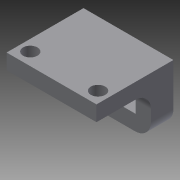
# Autodesk Inventor part: switch Holder
Saved by Autodesk Inventor 2014 (Build 180170000, 170)
## iProperties
Created: 2013-12-07
Part Number: switch Holder
Material: Generic
Document SubType Name: Modeling
Designer: Jesse Stevenson
Density: 1 g/cm^3
Appearance: Default
Author: Jesse Stevenson
Autodesk Inventor part; units mm, degrees
ref_plane "YZ Plane" through (0, 0, 0) normal (1, 0, 0) x (0, 1, 0)
ref_plane "XZ Plane" through (0, 0, 0) normal (0, 1, 0) x (-1, 0, 0)
ref_plane "XY Plane" through (0, 0, 0) normal (0, 0, 1) x (1, 0, 0)
sketch "Sketch1" plane through (0, 0, 0) normal (0, 0, 1) x (1, 0, 0)
  line L0 (0, 0) -> (29.2862, 0)
  line L1 (29.2862, 0) -> (29.2862, 13.716)
  line L2 (29.2862, 13.716) -> (0, 13.716)
  line L3 (0, 13.716) -> (0, 0)
  line L4 (14.6431, 13.716) -> (14.6431, 0) construction
  line L5 (0, 6.858) -> (29.2862, 6.858) construction
  line L6 (-7.62, -7.62) -> (36.9062, -7.62)
  line L7 (36.9062, -7.62) -> (36.9062, 21.336)
  line L8 (36.9062, 21.336) -> (-7.62, 21.336)
  line L9 (-7.62, 21.336) -> (-7.62, -7.62)
  line L10 (-7.62, -7.62) -> (36.9062, 21.336) construction
  line L11 (36.9062, -7.62) -> (-7.62, 21.336) construction
  point P0 (14.6431, 6.858)
  dimension "d0" = 29.2862
  dimension "d1" = 13.716
  dimension "d2" = 7.62
  dimension "d3" = 7.62
  constraints: 24 end point, 7 midpoint, 4 parallel, 2 horizontal, 2 perpendicular
  measures "d0" distance of L2.end L1.end
  measures "d1" distance of L1.end L0.end
  measures "d2" distance between parallel lines of L8 L2
  measures "d3" distance between parallel lines of L9 L3
extrude "Extrusion1" add sketch "Sketch1" along normal blind 11.1125
sketch "Sketch2" plane through (0, 0, 11.1125) normal (0, 0, 1) x (1, 0, 0)
  line L0 (0, 13.716) -> (29.2862, 13.716) projected
  line L1 (36.9062, -7.62) -> (36.9062, 21.336) projected
  line L2 (36.9062, 21.336) -> (-7.62, 21.336) projected
  line L3 (-7.62, 21.336) -> (-7.62, -7.62) projected
  line L4 (-7.62, 13.716) -> (0, 13.716)
  line L5 (29.2862, 13.716) -> (36.9062, 13.716)
  constraints: 4 end point, 2 perpendicular, 2 point on line
extrude "Extrusion2" add sketch "Sketch2" along normal blind 26.9875
sketch "Sketch3" plane through (0, 13.716, 0) normal (0, -1, 0) x (1, 0, 0)
  line L0 (36.9062, 11.1125) -> (36.9062, 38.1) projected
  line L1 (-7.62, 11.1125) -> (-7.62, 38.1) projected
  line L2 (-7.62, 31.837) -> (36.9062, 31.837) construction
  circle A0 centre (-2.1601, 31.837) radius 3.5719
  circle A1 centre (31.4297, 31.837) radius 3.5719
  dimension "d8" = 7.1437
  dimension "d9" = 7.1437
  constraints: 4 point on line, 2 centre point, 2 end point
  measures "d8" diameter of A0
  measures "d9" diameter of A1
extrude "Extrusion3" cut sketch "Sketch3" against normal through all
fillet "Fillet1" radius 7.9375 2 edges at (33.0962, 13.716, 11.1125) (-3.81, 13.716, 11.1125)
fillet "Fillet2" radius 7.9375 2 edges at (-7.62, -7.62, 5.5563) (36.9062, -7.62, 5.5563)
body "Solid1"
